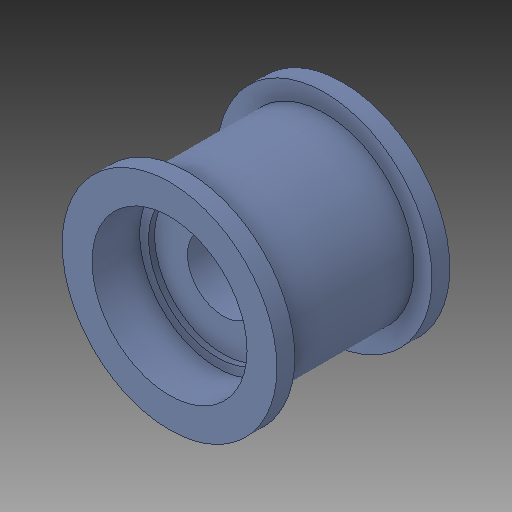
# Autodesk Inventor part: ABS Walze
Saved by Autodesk Inventor 2019 (Build 230136000, 136)
## iProperties
Created: 2021-11-05
Part Number: ABS Walze
Material: PC/ABS-Kunststoff
Document SubType Name: Modeling
Designer: Bergi
Density: 0.357273 g/cm^3
Appearance: Gummi - Blau
Mass: 4.21407 g
Surface Area: 71.4398 cm^2
Volume: 11.7951 cm^3
Author: Bergi
Autodesk Inventor part; units mm, degrees
ref_plane "YZ Plane" through (0, 0, 0) normal (1, 0, 0) x (0, 1, 0)
ref_plane "XZ Plane" through (0, 0, 0) normal (0, 1, 0) x (-1, 0, 0)
sketch "Skizze1" plane through (0, 0, 0) normal (0, 0, 1) x (1, 0, 0)
  circle A0 centre (0, 0) radius 15
  dimension "d0" = 30
  constraints: 1 centre point, 1 coincident
  measures "d0" diameter of A0
extrude "Extrusion1" add sketch "Skizze1" along normal blind 23
sketch "Skizze2" plane through (0, 0, 23) normal (0, 0, 1) x (1, 0, 0)
  circle A0 centre (0, 0) radius 18
  circle A1 centre (0, 0) radius 15 projected
  dimension "d3" = 3
  constraints: 1 centre point, 1 coincident
  measures "d3" radial gap between concentric circles of A0 A1
extrude "Extrusion2" add sketch "Skizze2" along normal blind 3 contours A0 | A1
ref_plane "Arbeitsebene1" through (0, 0, 11.5) normal (0, 0, -1) x (-1, 0, 0)
mirror "Spiegeln1" about plane through (0, 0, 11.5) normal (0, 0, -1) of "Extrusion2"
sketch "Skizze3" plane through (0, 0, 26) normal (0, 0, 1) x (1, 0, 0)
  circle A0 centre (0, 0) radius 13
  dimension "d6" = 26
  constraints: 1 centre point, 1 coincident
  measures "d6" diameter of A0
extrude "Extrusion3" cut sketch "Skizze3" against normal blind 8
sketch "Skizze4" plane through (0, 0, 18) normal (0, 0, 1) x (1, 0, 0)
  circle A0 centre (0, 0) radius 11.5
  circle A1 centre (0, 0) radius 13 projected
  dimension "d9" = 1.5
  constraints: 1 centre point, 1 coincident
  measures "d9" radial gap between concentric circles of A1 A0
extrude "Extrusion4" cut sketch "Skizze4" against normal blind 1 contours A0
mirror "Spiegeln2" about plane through (0, 0, 11.5) normal (0, 0, -1) of "Extrusion4", "Extrusion3"
sketch "Skizze5" plane through (0, 0, 17) normal (0, 0, 1) x (1, 0, 0)
  circle A0 centre (0, 0) radius 6
  dimension "d12" = 12
  constraints: 1 centre point, 1 coincident
  measures "d12" diameter of A0
extrude "Extrusion5" cut sketch "Skizze5" against normal through all
